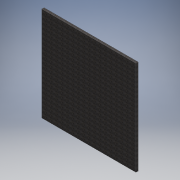
# Autodesk Inventor part: ConcreteFloor
Saved by Autodesk Inventor 2018 (Build 220112000, 112)
## iProperties
Created: 2017-09-19
Part Number: ConcreteFloor
Material: Concrete
Document SubType Name: Modeling
Designer: P136265
Density: 2.40731 g/cm^3
Appearance: Exposed Aggregate - Coarse
Author: P136265
Autodesk Inventor part; units mm, degrees
ref_plane "YZ Plane" through (0, 0, 0) normal (1, 0, 0) x (0, 1, 0)
ref_plane "XZ Plane" through (0, 0, 0) normal (0, 1, 0) x (-1, 0, 0)
ref_plane "XY Plane" through (0, 0, 0) normal (0, 0, 1) x (1, 0, 0)
sketch "Sketch1" plane through (0, 0, 0) normal (0, 0, 1) x (1, 0, 0)
  line L0 (-2000, -50) -> (2000, -50)
  line L1 (2000, -50) -> (2000, 50)
  line L2 (2000, 50) -> (-2000, 50)
  line L3 (-2000, 50) -> (-2000, -50)
  line L4 (-2000, -50) -> (2000, 50) construction
  line L5 (2000, -50) -> (-2000, 50) construction
  point P0 (0, 0)
  dimension "d0" = 4000
  dimension "d1" = 100
  constraints: 12 end point, 2 midpoint, 2 parallel, 1 horizontal, 1 perpendicular
  measures "d0" distance of L2.end L1.end
  measures "d1" distance of L1.end L0.end
extrude "Extrusion1" add sketch "Sketch1" along normal mid plane 4000
body "Solid1"
